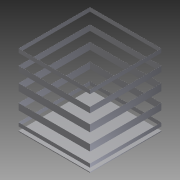
# Autodesk Inventor part: Cage
Saved by Autodesk Inventor 2011 SP2 (Build 150309200, 309)
## iProperties
Created: 2015-10-15
Part Number: Cage
Document SubType Name: Modeling
Designer: Ernest
Density: 1 g/cm^3
Mass: 92.0668 g
Surface Area: 2009.9 cm^2
Volume: 92.0668 cm^3
Author: Ernest
Autodesk Inventor part; units mm, degrees
ref_plane "YZ Plane" through (0, 0, 0) normal (1, 0, 0) x (0, 1, 0)
ref_plane "XZ Plane" through (0, 0, 0) normal (0, 1, 0) x (-1, 0, 0)
ref_plane "XY Plane" through (0, 0, 0) normal (0, 0, 1) x (1, 0, 0)
sketch "Sketch1" plane through (0, 0, 0) normal (0, 0, 1) x (1, 0, 0)
  line L0 (0, 0) -> (200, 0)
  line L1 (200, 0) -> (200, 200)
  line L2 (200, 200) -> (0, 200)
  line L3 (0, 200) -> (0, 0)
  dimension "d0" = 200
  dimension "d1" = 200
  constraints: 8 end point, 2 parallel, 1 horizontal, 1 perpendicular
  measures "d0" distance of L2.end L1.end
  measures "d1" distance of L1.end L0.end
extrude "Extrusion1" add sketch "Sketch1" along normal blind 2
sketch "Sketch2" plane through (0, 0, 2) normal (0, 0, 1) x (1, 0, 0)
  line L0 (0, 0) -> (0, 200) projected
  line L1 (200, 0) -> (0, 0) projected
  line L2 (200, 200) -> (200, 0) projected
  line L3 (0, 200) -> (200, 200) projected
  line L4 (200, 0) -> (0, 0)
  line L5 (0, 0) -> (0, 200)
  line L6 (0, 200) -> (200, 200)
  line L7 (200, 200) -> (200, 0)
  line L8 (200.2, -0.2) -> (-0.2, -0.2)
  line L9 (-0.2, -0.2) -> (-0.2, 200.2)
  line L10 (-0.2, 200.2) -> (200.2, 200.2)
  line L11 (200.2, 200.2) -> (200.2, -0.2)
  dimension "d4" = 0.2
  dimension "d5" = 0.2
  dimension "d6" = 0.2
  dimension "d7" = 0.2
  constraints: 16 end point, 4 parallel, 2 horizontal, 2 perpendicular
  measures "d4" distance between parallel lines of L4 L8
  measures "d5" distance between parallel lines of L11 L2
  measures "d6" distance between parallel lines of L9 L0
  measures "d7" distance between parallel lines of L3 L10
extrude "Extrusion2" add sketch "Sketch2" along normal blind 200 and the other way blind 2
sketch "Sketch3" plane through (-0.2, 200.2, 202) normal (0, 1, 0) x (1, 0, 0)
  line L0 (223.7217, 10.8439) -> (-23.2228, 10.8439)
  line L1 (-23.2228, 10.8439) -> (-23.2228, 41.9406)
  line L2 (-23.2228, 41.9406) -> (223.7217, 41.9406)
  line L3 (223.7217, 41.9406) -> (223.7217, 10.8439)
  line L4 (223.7217, 57.4889) -> (-23.2228, 57.4889)
  line L5 (-23.2228, 57.4889) -> (-23.2228, 84.4699)
  line L6 (-23.2228, 84.4699) -> (223.7217, 84.4699)
  line L7 (223.7217, 84.4699) -> (223.7217, 57.4889)
  line L8 (223.7217, 103.6767) -> (-23.2228, 103.6767)
  line L9 (-23.2228, 103.6767) -> (-23.2228, 132.4869)
  line L10 (-23.2228, 132.4869) -> (223.7217, 132.4869)
  line L11 (223.7217, 132.4869) -> (223.7217, 103.6767)
  line L12 (223.7217, 150.3218) -> (-23.2228, 150.3218)
  line L13 (-23.2228, 150.3218) -> (-23.2228, 179.5893)
  line L14 (-23.2228, 179.5893) -> (223.7217, 179.5893)
  line L15 (223.7217, 179.5893) -> (223.7217, 150.3218)
  line L16 (223.7217, 189.4978) -> (-23.2228, 189.4978)
  line L17 (-23.2228, 189.4978) -> (-23.2228, 200)
  line L18 (-23.2228, 200) -> (223.7217, 200)
  line L19 (223.7217, 200) -> (223.7217, 189.4978)
  point P0 (0.2, 202)
  constraints: 40 end point, 10 parallel, 5 horizontal, 5 perpendicular
extrude "Extrusion3" cut sketch "Sketch3" against normal through all
body "Solid1"
